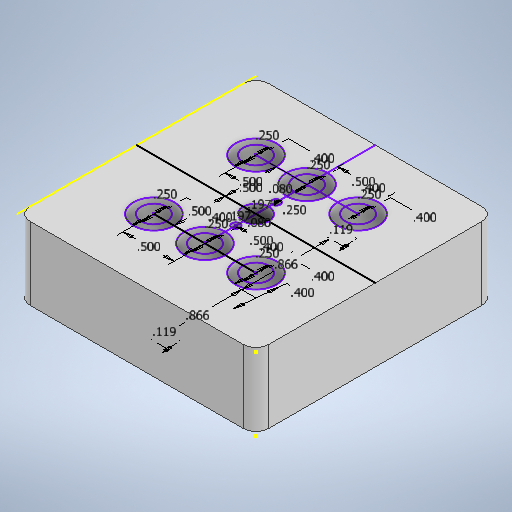
# Autodesk Inventor part: LNR25MtoPolarisAdapter
Saved by Autodesk Inventor 2025.2 (Build 292293000, 293)
## iProperties
Created: 2026-01-16
Part Number: LNR25MtoPolarisAdapter
Material: Generic
Document SubType Name: Modeling
Designer: monolithic
Density: 1 g/cm^3
Appearance: Default
Author: monolithic
Autodesk Inventor part; units mm, degrees
ref_plane "YZ Plane" through (0, 0, 0) normal (1, 0, 0) x (0, 1, 0)
ref_plane "XZ Plane" through (0, 0, 0) normal (0, 1, 0) x (-1, 0, 0)
ref_plane "XY Plane" through (0, 0, 0) normal (0, 0, 1) x (1, 0, 0)
sketch "Sketch1" plane through (0, 0, 0) normal (0, 1, 0) x (-1, 0, 0)
  line L0 (0, 0) -> (59.4, 0)
  line L1 (59.4, 0) -> (59.4, -59.4)
  line L2 (59.4, -59.4) -> (0, -59.4)
  line L3 (0, -59.4) -> (0, 0)
  dimension "d0" = 59.4
  dimension "d1" = 59.4
  constraints: 8 end point, 2 parallel, 1 horizontal, 1 perpendicular
  measures "d0" distance of L1.end L2.end
  measures "d1" distance of L0.end L1.end
extrude "Extrusion1" add sketch "Sketch1" along normal blind 18.1
sketch "Sketch2" plane through (0, 18.1, 0) normal (0, 1, 0) x (1, 0, 0)
  line L0 (-59.4, 59.4) -> (-59.4, 0) projected
  line L1 (-59.4, 29.7) -> (0, 29.7)
  line L2 (-29.7, 29.7) -> (-29.7, 59.4)
  line L3 (-29.7, 29.7) -> (-29.7, 17)
  circle A0 centre (-29.7, 17) radius 5.08
  line L4 (-29.7, 17) -> (-42.4, 17)
  line L5 (-29.7, 17) -> (-17, 17)
  circle A1 centre (-42.4, 17) radius 5.08
  circle A2 centre (-17, 17) radius 5.08
  line L6 (-29.7, 29.7) -> (-29.7, 42.4)
  circle A3 centre (-29.7, 42.4) radius 5.08
  line L7 (-29.7, 42.4) -> (-42.4, 42.4)
  line L8 (-29.7, 42.4) -> (-17, 42.4)
  circle A4 centre (-42.4, 42.4) radius 5.08
  circle A5 centre (-17, 42.4) radius 5.08
  circle A6 centre (-29.7, 17) radius 3.175
  circle A7 centre (-42.4, 17) radius 3.175
  circle A8 centre (-17, 17) radius 3.175
  circle A9 centre (-29.7, 42.4) radius 3.175
  circle A10 centre (-42.4, 42.4) radius 3.175
  circle A11 centre (-17, 42.4) radius 3.175
  circle A12 centre (-29.7, 29.7) radius 3.175
  line L9 (-29.7, 29.7) -> (-29.7, 34.704)
  line L10 (-29.7, 29.7) -> (-29.7, 24.696)
  circle A13 centre (-29.7, 24.696) radius 1.0125
  circle A14 centre (-29.7, 34.704) radius 1.0125
  point P0 (0, 0)
  dimension "d4" = 12.7
  dimension "d5" = 10.16
  dimension "d6" = 12.7
  dimension "d7" = 12.7
  dimension "d8" = 10.16
  dimension "d9" = 10.16
  dimension "d10" = 12.7
  dimension "d11" = 10.16
  dimension "d12" = 12.7
  dimension "d13" = 12.7
  dimension "d14" = 10.16
  dimension "d15" = 10.16
  dimension "d16" = 6.35
  dimension "d17" = 6.35
  dimension "d18" = 6.35
  dimension "d19" = 6.35
  dimension "d20" = 6.35
  dimension "d21" = 6.35
  dimension "d22" = 6.35
  dimension "d23" = 5.004
  dimension "d24" = 5.004
  dimension "d25" = 2.025
  dimension "d26" = 2.025
  constraints: 20 end point, 15 centre point, 7 coincident, 5 horizontal, 3 point on line, 2 midpoint, 2 vertical
  measures "d4" distance of L2.start L3.end
  measures "d5" diameter of A0
  measures "d6" distance of L4.start L4.end
  measures "d7" distance of L4.start L5.end
  measures "d8" diameter of A1
  measures "d9" diameter of A2
  measures "d10" distance of L2.start L6.end
  measures "d11" diameter of A3
  measures "d12" distance of L7.start L7.end
  measures "d13" distance of L7.start L8.end
  measures "d14" diameter of A4
  measures "d15" diameter of A5
  measures "d16" diameter of A6
  measures "d17" diameter of A7
  measures "d18" diameter of A8
  measures "d19" diameter of A9
  measures "d20" diameter of A10
  measures "d21" diameter of A11
  measures "d22" diameter of A12
  measures "d23" distance of L9.start L9.end
  measures "d24" distance of L9.start L10.end
  measures "d25" diameter of A13
  measures "d26" diameter of A14
extrude "Extrusion2" cut sketch "Sketch2" against normal blind 38.1 contours L2 A12 L1 | L3 A12 L1 | L1 A12 L2 | L1 A12 L3 | A8 | A7 | A10 | A11 | A9 L7 L2 | L2 L8 A9 | A6 L5 L3 | L3 L4 A6 | L7 A9 L2 | L2 A9 L8 | L5 A6 L4
extrude "Extrusion3" cut sketch "Sketch2" against normal blind 7.62 contours A8 | A2 | A7 | A1 | A0 L5 A6 L3 | L3 A6 L4 A0 | A4 | A11 | A5 | A3 L7 A9 L2 | L2 A9 L8 A3 | A9 L7 L2 | L2 L8 A9 | A3 L2 A9 L7 | L8 A9 L2 A3 | A6 L5 L3 | L3 L4 A6 | A0 L4 A6 L5 | L7 A9 L2 | L2 A9 L8 | L5 A6 L4
extrude "Extrusion4" cut sketch "Sketch2" against normal blind 4.445 contours A13 L3 | L3 A13 | A14 L2 | L2 A14
sketch "Sketch3" plane through (0, 0, 0) normal (0, -1, 0) x (1, 0, 0)
  circle A0 centre (-29.7, -29.7) radius 3.175 projected
  line L0 (-29.7, -29.7) -> (-29.7, -51.7)
  line L1 (-29.7, -29.7) -> (-29.7, -7.7)
  circle A1 centre (-29.7, -7.7) radius 1.5125
  circle A2 centre (-29.7, -51.7) radius 1.5125
  circle A3 centre (-29.7, -29.7) radius 5.08
  point P0 (0, 0)
  dimension "d33" = 22
  dimension "d34" = 22
  dimension "d35" = 3.025
  dimension "d36" = 3.025
  dimension "d37" = 10.16
  constraints: 4 end point, 3 centre point, 3 coincident, 2 vertical
  measures "d33" distance of L0.start L0.end
  measures "d34" distance of L0.start L1.end
  measures "d35" diameter of A1
  measures "d36" diameter of A2
  measures "d37" diameter of A3
extrude "Extrusion5" cut sketch "Sketch3" against normal blind 4.445 contours A1 | A2
extrude "Extrusion6" cut sketch "Sketch3" against normal blind 7.62 contours A0 L0 L1 | A0 L1 A3 L0 | L1 L0 A0 | A0 L0 A3 L1
fillet "Fillet1" radius 3.175 4 edges at (0, 9.05, -59.4) (0, 9.05, 0) (-59.4, 9.05, 0) (-59.4, 9.05, -59.4)
body "Solid1"
